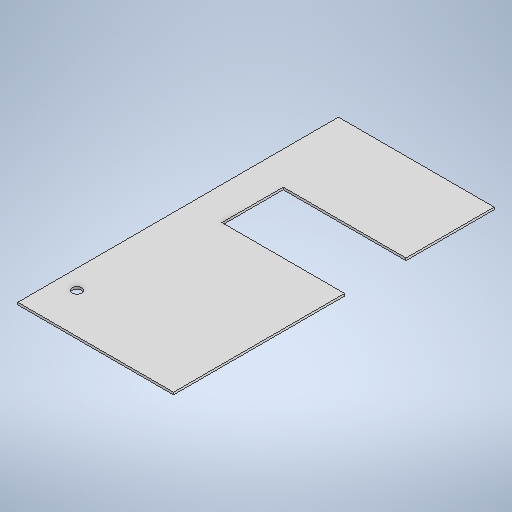
# Autodesk Inventor part: scina_fronotwa
Saved by Autodesk Inventor 2026.2 (Build 302298010, 298A)
## iProperties
Created: 2026-04-29
Part Number: scina_fronotwa
Material: Ogólny
Document SubType Name: Modeling
Designer: Patryk
Density: 1 g/cm^3
Appearance: Domyślna
Author: Patryk
Autodesk Inventor part; units mm, degrees
ref_plane "YZ Plane" through (0, 0, 0) normal (1, 0, 0) x (0, 1, 0)
ref_plane "XZ Plane" through (0, 0, 0) normal (0, 1, 0) x (-1, 0, 0)
ref_plane "XY Plane" through (0, 0, 0) normal (0, 0, 1) x (1, 0, 0)
sketch "Szkic1" plane through (0, 0, 0) normal (0, 1, 0) x (-1, 0, 0)
  line L0 (-101.5, -209) -> (101.5, -209)
  line L1 (101.5, -209) -> (101.5, 209)
  line L2 (101.5, 209) -> (-101.5, 209)
  line L3 (-101.5, 209) -> (-101.5, -209)
  line L4 (-101.5, -209) -> (101.5, 209) construction
  line L5 (101.5, -209) -> (-101.5, 209) construction
  line L6 (-101.5, -94) -> (58.5, -94)
  line L7 (58.5, -94) -> (58.5, -14)
  line L8 (58.5, -14) -> (-101.5, -14)
  line L9 (-101.5, -14) -> (-101.5, -94)
  circle A0 centre (76.5, 157) radius 6.1
  point P0 (0, 0)
  dimension "d0" = 203
  dimension "d1" = 418
  dimension "d2" = 160
  dimension "d3" = 80
  dimension "d4" = 115
  dimension "d5" = 12.2
  dimension "d6" = 25
  dimension "d7" = 52
  constraints: 20 end point, 4 parallel, 2 horizontal, 2 midpoint, 2 perpendicular, 1 centre point, 1 point on line
  measures "d0" distance of L2.end L1.end
  measures "d1" distance of L1.end L0.end
  measures "d2" distance of L8.end L7.end
  measures "d3" distance of L7.end L6.end
  measures "d4" distance between parallel lines of L0 L6
  measures "d5" diameter of A0
  measures "d6" distance from line of L1 A0.centre
  measures "d7" distance from line of L2 A0.centre
extrude "Wyciągnięcie proste1" add sketch "Szkic1" along normal mid plane 3 contours L3 L6 L7 L8 L2 L1 L0
